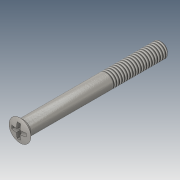
# Autodesk Inventor part: Parafuso do Braço (2)
Saved by Autodesk Inventor 2016 (Build 200138000, 138)
## iProperties
Created: 2018-12-08
Part Number: Parafuso do Braço (2)
Material: Generic
Document SubType Name: Modeling
Designer: Pedro Mendonça
Density: 1 g/cm^3
Appearance: Galvanized
Author: Pedro Mendonça
Autodesk Inventor part; units mm, degrees
ref_plane "YZ Plane" through (0, 0, 0) normal (1, 0, 0) x (0, 1, 0)
ref_plane "XZ Plane" through (0, 0, 0) normal (0, 1, 0) x (-1, 0, 0)
sketch "Sketch1" plane through (0, 0, 0) normal (1, 0, 0) x (0, 1, 0)
  circle A0 centre (0, 0) radius 2.05
  dimension "d0" = 4.1
  constraints: 1 centre point, 1 coincident
  measures "d0" diameter of A0
extrude "Extrusion1" add sketch "Sketch1" against normal blind 38
ref_plane "Work Plane1" through (1, 0, 0) normal (1, 0, 0) x (0, 0, -1)
sketch "Sketch2" plane through (1, 0, 0) normal (1, 0, 0) x (0, 0, -1)
  circle A0 centre (0, 0) radius 3
  dimension "d4" = 6
  constraints: 1 centre point, 1 coincident
  measures "d4" diameter of A0
loft "Loft1" add profiles "Sketch2" section 1 edges at (0, -2.05, 0)
sketch "Sketch3" plane through (0, 0, 0) normal (0, 1, 0) x (-1, 0, 0)
  line L0 (-1, -3) -> (-1, 3) projected
  line L1 (-1, 3) -> (-1, 0)
  line L2 (-1, 0) -> (-1.5, 0)
  arc A0 (-1, 3) -> (-1.5, 0) centre (7.75, 0) ccw
  point P0 (0, 0)
  dimension "d9" = 0.5
  constraints: 4 end point, 2 point on circle, 1 centre point, 1 midpoint, 1 perpendicular
  measures "d9" distance of L2.end L1.end
revolve "Revolution1" add sketch "Sketch3" angle 360 about axis through (1, 0, 0) along (1, 0, 0)
ref_plane "Work Plane2" through (1.5, 0, 0) normal (1, 0, 0) x (0, 0, -1)
sketch "Sketch4" plane through (1.5, 0, 0) normal (1, 0, 0) x (0, 0, -1)
  line L0 (2, 0.5) -> (2, -0.5)
  line L1 (-2, -0.5) -> (-2, 0.5)
  line L2 (-0.5, 2) -> (0.5, 2)
  line L3 (0.5, -2) -> (-0.5, -2)
  line L4 (2, -0.5) -> (0.5, -0.5)
  line L5 (-0.5, -0.5) -> (-2, -0.5)
  line L6 (-0.5, -2) -> (-0.5, -0.5)
  line L7 (-0.5, 0.5) -> (-0.5, 2)
  line L8 (-2, 0.5) -> (-0.5, 0.5)
  line L9 (0.5, 0.5) -> (2, 0.5)
  line L10 (0.5, 2) -> (0.5, 0.5)
  line L11 (0.5, -0.5) -> (0.5, -2)
  dimension "d12" = 4
  dimension "d13" = 1
  dimension "d14" = 1
  dimension "d15" = 4
  constraints: 24 end point, 10 parallel, 4 perpendicular, 3 horizontal
  measures "d12" distance of L0.end L1.start
  measures "d13" distance of L0.start L0.end
  measures "d14" distance of L3.start L3.end
  measures "d15" distance of L2.end L3.start
extrude "Extrusion2" cut sketch "Sketch4" against normal blind 1 draft -10
chamfer "Chamfer1" distance 0.5 angle 45 1 edges at (-38, -2.05, 0)
thread "Thread1" size "M4.5x0.75" class "6g" standard "ANSI Metric M Profile" length 15
body "Solid1"
